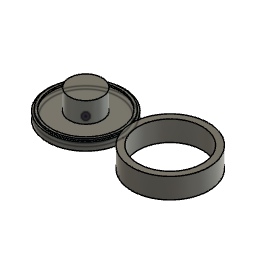
Rosita (Molde rueda siliciona) v3 (nose si es el molde) (Autodesk Fusion 360 design; units mm, degrees)
Autodesk Fusion 360 part; units mm, degrees
note: some values were not read from the file. Chosen so that the rebuilt part matches the saved one: which bodies a step acts on.
sketch "Boceto1" plane through (0, 0, 0) normal (0, 1, 0) x (1, 0, 0)
  circle A0 centre (0, 0) radius 10.5
  circle A1 centre (0, 0) radius 20.5
  circle A2 centre (0, 0) radius 24.5
  dimension "d1" = 21
  dimension "d3" = 10
  dimension "d4" = 14
  constraint coincident A0.centre A1.centre
  measures "d1" diameter of A0
ref_plane "PlanoDeObra1" through (0, 2, 0) normal (0, 1, 0) x (1, 0, 0)
sketch "Boceto2" plane through (0, 2, 0) normal (0, 1, 0) x (1, 0, 0)
  circle A0 centre (0, 0) radius 21.3
  circle A1 centre (0, 0) radius 23.8
  dimension "d12" = 42.6
  dimension "d13" = 47.6
  constraint coincident A0.centre A1.centre
  constraint concentric A0 A1
  measures "d12" diameter of A0
  measures "d13" diameter of A1
combine "Combinar1" [no effect]
extrude "Extruir12" add sketch "Boceto1" along normal blind 2 contours A0 | A1 | A2 makes body 1
extrude "Extruir13" add sketch "Boceto1" along normal blind 15 bodies 1
extrude "Extruir14" cut sketch "Boceto2" along normal blind 1 bodies 1
split "Dividir2" by plane through (0, 2, 0) normal (0, 1, 0) bodies 1 makes body 2 at (24.3783, 6.3333, -2.4394) makes body 3 at (10.4478, 6.3333, -1.0455)
extrude "Extruir15" add sketch "Boceto2" along normal blind 1 bodies 1
combine "Combinar2" operation add target body 1 tool bodies 3
move_body "Desplazar1" bodies 2 to x (1, 0, 0) y (0, 1, 0) z (0, 0, 1) at (54, -2, 0)
extrude "Extruir16" add 1 faces at (8.8365, 0, -2.1715) along direction (0, -1, 0) blind 3 on bodies 1 bodies 1
move_body "Desplazar2" bodies 1 to x (1, 0, 0) y (0, 1, 0) z (0, 0, 1) at (0, 3, 0)
move_face "CarasDesfase1" offset -0.5 2 faces at (23.6817, 5.3333, 2.3697) (21.1942, 5.3333, 2.1208) on bodies 1
equation "d1 = 10.5 mm + 10.5 mm"
equation "d12 = 47.60 mm - 5 mm"
equation "d13 = 17 mm + 10.5 mm + 20.1 mm"
named bodies: "Base", "Tapa"
